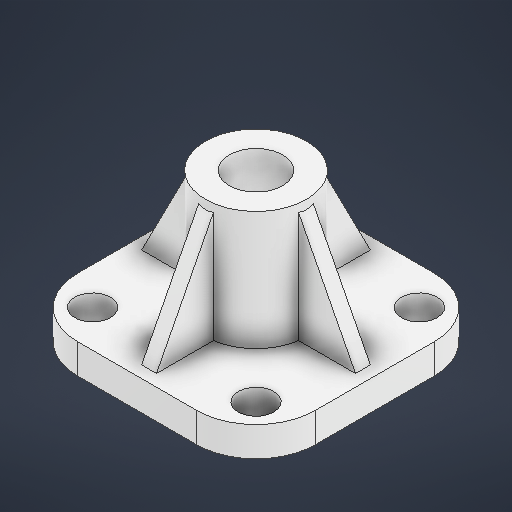
# Autodesk Inventor part: Flanged Support
Saved by Autodesk Inventor 2026.2 (Build 302298000, 298)
## iProperties
Created: 2026-02-13
Part Number: Flanged Support
Material: Generic
Document SubType Name: Modeling
Designer: chuan
Density: 1 g/cm^3
Appearance: Snow
Author: chuan
Autodesk Inventor part; units mm, degrees
ref_plane "YZ Plane" through (0, 0, 0) normal (1, 0, 0) x (0, 1, 0)
ref_plane "XZ Plane" through (0, 0, 0) normal (0, 1, 0) x (-1, 0, 0)
ref_plane "XY Plane" through (0, 0, 0) normal (0, 0, 1) x (1, 0, 0)
sketch "Sketch1" plane through (0, 0, 0) normal (0, 1, 0) x (-1, 0, 0)
  line L0 (-40, 40) -> (40, 40)
  line L1 (40, 40) -> (40, -40)
  line L2 (40, -40) -> (-40, -40)
  line L3 (-40, -40) -> (-40, 40)
  line L4 (-40, 40) -> (40, -40) construction
  line L5 (40, 40) -> (-40, -40) construction
  point P0 (0, 0)
  dimension "d0" = 80
  dimension "d1" = 80
  constraints: 12 end point, 2 midpoint, 2 parallel, 1 horizontal, 1 perpendicular
  measures "d0" distance of L1.end L2.end
  measures "d1" distance of L0.end L1.end
extrude "Extrusion1" add sketch "Sketch1" along normal blind 10
fillet "Fillet1" radius 20 4 edges at (40, 5, 40) (-40, 5, 40) (40, 5, -40) (-40, 5, -40)
sketch "Sketch2" plane through (0, 10, 0) normal (0, 1, 0) x (1, 0, 0)
  circle A0 centre (-27.5, -27.5) radius 6
  circle A1 centre (-27.5, 27.5) radius 6
  circle A2 centre (27.5, -27.5) radius 6
  circle A3 centre (27.5, 27.5) radius 6
  point P0 (0, 0)
  dimension "d5" = 12
  dimension "d6" = 55
  dimension "d7" = 55
  dimension "d8" = 27.5
  dimension "d9" = 27.5
  constraints: 4 centre point, 3 equal radius, 2 horizontal alignment, 2 vertical alignment
  measures "d5" diameter of A1
  measures "d6" distance of A3.centre A1.centre
  measures "d7" distance of A0.centre A1.centre
  measures "d8" horizontal distance of point (0, 0) A0.centre
  measures "d9" horizontal distance of point (0, 0) A3.centre
extrude "Extrusion2" cut sketch "Sketch2" against normal through all
sketch "Sketch3" plane through (0, 10, 0) normal (0, 1, 0) x (1, 0, 0)
  circle A0 centre (0, 0) radius 9
  circle A1 centre (0, 0) radius 17
  dimension "d12" = 18
  dimension "d13" = 34
  constraints: 2 centre point, 2 coincident
  measures "d12" diameter of A0
  measures "d13" diameter of A1
extrude "Extrusion3" add sketch "Sketch3" along normal blind 40
sketch "Sketch4" plane through (0, 0, 0) normal (0, 0, 1) x (1, 0, 0)
  line L0 (21.5, 10) -> (33.5, 10) projected
  line L1 (36, 10) -> (17, 47)
  line L2 (40, 10) -> (40, 0) projected
  point P0 (0, 0)
  dimension "d16" = 4
  dimension "d17" = 37
  constraints: 2 end point, 1 point on line
  measures "d16" distance from line of L2 L1.start
  measures "d17" vertical distance of L1.end L1.start
extrude "Rib1" add sketch "Sketch4" along normal mid plane 5 rib yes fills toward (26.4555, 28.4772) open curves L1
pattern_circular "Circular Pattern1" count 4 over 360 about axis through (0, 10, 0) along (0, 1, 0) of "Rib1"
extrude "Extrusion4" cut sketch "Sketch3" against normal through all contours A0
body "Solid1"
